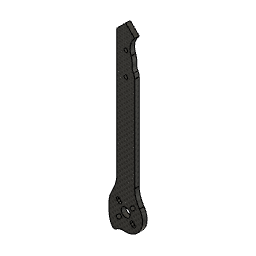
frame_arm_4mm (Autodesk Fusion 360 design; units mm, degrees)
Autodesk Fusion 360 part; units mm, degrees
sketch "Sketch3" plane through (0, 0, 0) normal (0, 0, 1) x (1, 0, 0)
  circle A0 centre (0.0083, -64.5282) radius 4.05
  circle A1 centre (0.0083, -64.5282) radius 8.75 construction
  line L0 (0.0083, -64.5282) -> (6.1955, -58.341) construction
  line L1 (0.0083, -64.5282) -> (8.7583, -64.5282) construction
  line L2 (6.4784, -60.1795) -> (8.034, -58.6238)
  arc A2 (8.034, -58.6238) -> (5.9127, -56.5025) centre (6.9733, -57.5632) ccw
  line L3 (5.9127, -56.5025) -> (4.357, -58.0581)
  arc A3 (4.357, -58.0581) -> (6.4784, -60.1795) centre (5.4177, -59.1188) ccw
  line L4 (4.357, -60.1795) -> (8.034, -56.5025) construction
  line L5 (4.357, -60.1795) -> (7.9558, -60.1795) construction
  line L6 (-4.3404, -58.0581) -> (-5.896, -56.5025)
  line L7 (-8.0173, -58.6238) -> (-6.4617, -60.1795)
  arc A4 (-6.4617, -60.1795) -> (-4.3404, -58.0581) centre (-5.401, -59.1188) ccw
  line L8 (-4.3404, -60.1795) -> (-8.0173, -56.5025) construction
  arc A5 (-5.896, -56.5025) -> (-8.0173, -58.6238) centre (-6.9567, -57.5632) ccw
  line L9 (-6.4617, -68.8769) -> (-8.0173, -70.4325)
  line L10 (-5.896, -72.5538) -> (-4.3404, -70.9982)
  arc A6 (-4.3404, -70.9982) -> (-6.4617, -68.8769) centre (-5.401, -69.9375) ccw
  line L11 (-4.3404, -68.8769) -> (-8.0173, -72.5538) construction
  arc A7 (-8.0173, -70.4325) -> (-5.896, -72.5538) centre (-6.9567, -71.4932) ccw
  line L12 (4.357, -70.9982) -> (5.9127, -72.5538)
  line L13 (8.034, -70.4325) -> (6.4784, -68.8769)
  arc A8 (6.4784, -68.8769) -> (4.357, -70.9982) centre (5.4177, -69.9375) ccw
  line L14 (4.357, -68.8769) -> (8.034, -72.5538) construction
  arc A9 (5.9127, -72.5538) -> (8.034, -70.4325) centre (6.9733, -71.4932) ccw
  circle A10 centre (0.0083, -64.5282) radius 15.1
  line L15 (-8.8515, -81.7805) -> (-9.2245, -82.0856)
  line L16 (-11.4526, -81.7512) -> (-11.2758, -81.9426)
  arc A11 (-1.4818, -79.5545) -> (-8.8515, -81.7805) centre (-2.4756, -89.5764) ccw
  line L17 (0.0083, -64.5282) -> (-15.0917, -64.5282) construction
  spline S0 degree 5 poles (-11.4526, -81.7512) (-11.5434, -81.653) (-11.7181, -81.4571) (-11.959, -81.1655) (-12.2453, -80.7768) (-12.5785, -80.2658) (-12.9207, -79.695) (-13.2839, -79.026) (-13.6569, -78.2216) (-14.017, -77.2506) (-14.3381, -76.0931) (-14.6006, -74.7468) (-14.7984, -73.2325) (-14.9351, -71.5854) (-15.0206, -69.8489) (-15.0676, -68.0675) (-15.0846, -66.6385) (-15.0904, -65.5777) (-15.0917, -64.8769) (-15.0917, -64.5282) knots 0 0 0 0 0 0 0.066667 0.133333 0.2 0.266667 0.333333 0.4 0.466667 0.533333 0.6 0.666667 0.733333 0.8 0.866667 0.933333 1 1 1 1 1 1
  arc A12 (-11.2758, -81.9426) -> (-9.2245, -82.0856) centre (-10.1742, -80.9245) ccw
  line L18 (0, 0) -> (-8.1, 0) construction
  line L19 (-8.1, 0) -> (-8.1, 74.424)
  line L20 (-8.1, 0) -> (-8.1, -40.576)
  spline S1 degree 5 poles (-15.0917, -64.5282) (-15.0917, -64.2457) (-15.0821, -63.684) (-15.0388, -62.8507) (-14.9249, -61.7598) (-14.6973, -60.4356) (-14.3963, -59.1591) (-14.0349, -57.9381) (-13.626, -56.7786) (-13.1797, -55.6822) (-12.7048, -54.6455) (-12.2091, -53.6579) (-11.7011, -52.7014) (-11.1912, -51.7478) (-10.6919, -50.7589) (-10.216, -49.6979) (-9.7711, -48.5441) (-9.3608, -47.2978) (-8.9724, -46.0117) (-8.6188, -44.7062) (-8.3284, -43.3781) (-8.1734, -42.2856) (-8.1133, -41.4415) (-8.1, -40.8665) (-8.1, -40.576) knots 0 0 0 0 0 0 0.05 0.1 0.15 0.2 0.25 0.3 0.35 0.4 0.45 0.5 0.55 0.6 0.65 0.7 0.75 0.8 0.85 0.9 0.95 1 1 1 1 1 1
  line L21 (-10.3594, -50.3117) -> (-8.6813, -45.2176)
  line L22 (-8.1, 74.424) -> (-0.039, 82.4851)
  line L23 (-8.1, 74.424) -> (3.05, 74.424) construction
  line L24 (-0.039, 82.4851) -> (8.022, 74.424)
  line L25 (-0.039, 82.4851) -> (11.1696, 82.4851) construction
  line L26 (8.022, 74.424) -> (18.0806, 64.3654) construction
  arc A13 (8.022, 74.424) -> (4.8004, 59.2677) centre (18.0806, 64.3654) ccw
  line L27 (18.0806, 64.3654) -> (8.022, 74.424) construction
  line L28 (18.0806, 64.3654) -> (4.8004, 59.2677) construction
  spline S2 degree 5 poles (4.8004, 59.2677) (4.8494, 59.1404) (4.9423, 58.8866) (5.0666, 58.5087) (5.2043, 58.0107) (5.3432, 57.4017) (5.4642, 56.809) (5.5795, 56.2321) (5.6934, 55.6644) (5.7974, 55.0914) (5.8765, 54.4957) (5.916, 53.8616) (5.9073, 53.1806) (5.8552, 52.4567) (5.782, 51.71) (5.7191, 50.9686) (5.6999, 50.2615) (5.7511, 49.6111) (5.8867, 49.0267) (6.0971, 48.4946) (6.3562, 47.9853) (6.5772, 47.5687) (6.7385, 47.238) (6.8424, 47.0077) (6.8934, 46.89) knots 0 0 0 0 0 0 0.05 0.1 0.15 0.2 0.25 0.3 0.35 0.4 0.45 0.5 0.55 0.6 0.65 0.7 0.75 0.8 0.85 0.9 0.95 1 1 1 1 1 1
  line L29 (4.1339, 60.9997) -> (5.467, 57.5357) construction
  line L30 (6.1548, 48.5926) -> (7.632, 45.1875) construction
  circle A14 centre (-0.1012, 42.8053) radius 8.1 construction
  circle A15 centre (0, 61.4851) radius 1.6
  circle A16 centre (0, 40.6251) radius 1.6
  circle A17 centre (-0.1012, 42.8053) radius 8.1
  line L31 (0, 0) -> (0, 40.6251)
  line L32 (-0.1012, 42.8053) -> (7.9988, 42.8053) construction
  line L33 (7.9988, 42.8053) -> (7.9988, -42.1947)
  arc A18 (7.9988, -42.1947) -> (12.3295, -55.799) centre (31.5321, -42.1947) ccw
  point P0 (6.1955, -58.341)
  point P1 (-6.1789, -58.341)
  point P2 (-6.1789, -58.341)
  point P3 (-6.1789, -70.7154)
  point P4 (-6.1789, -70.7154)
  point P5 (6.1955, -70.7154)
  point P6 (6.1955, -70.7154)
  point P7 (-12.7288, -80.0085)
  point P8 (-14.2896, -76.1896)
  point P9 (-13.921, -57.6445)
  point P10 (-11.7496, -52.7944)
  point P11 (-9.5204, -47.7647)
  point P12 (5.9008, 53.2841)
  point P13 (5.5742, 56.2588)
  point P14 (5.7979, 49.475)
  dimension "d1" = 8.1
  dimension "d2" = 17.5
  dimension "d3" = 45
  dimension "d4" = 5.2
  dimension "d5" = 45
  dimension "d6" = 3
  dimension "d8" = 360
  dimension "d9" = 30.2
  dimension "d10" = 1.5
  dimension "d11" = 8.1
  dimension "d12" = 115
  dimension "d13" = 45
  dimension "d14" = 11.4
  dimension "d15" = 45
  dimension "d16" = 11.4
  dimension "d17" = 14.225
  dimension "d18" = 66
  dimension "d19" = 3.2
  dimension "d20" = 21
  dimension "d21" = 3.2
  dimension "d22" = 20.86
  dimension "d23" = 16.2
  dimension "d24" = 85
  constraint concentric A0 A1
  constraint horizontal L1
  constraint coincident A0.centre A1.centre
  constraint coincident A1 P0
  constraint tangent L2 A2
  constraint tangent A2 L3
  constraint parallel L2 L3
  constraint tangent L3 A3
  constraint tangent L2 A3
  constraint midpoint A3 L4.start
  constraint midpoint A2 L4.end
  constraint coincident L0 L4.start
  constraint parallel L0 L4
  constraint midpoint L4 P0
  constraint coincident P0 L0.end
  constraint concentric A1 A10
  constraint tangent L15 A11
  constraint coincident A10 A11.start
  constraint tangent A10 A11
  constraint coincident A10 L17.end
  constraint parallel L1 L17
  constraint tangent A10 S0
  constraint tangent L15 A12
  constraint tangent L16 A12
  constraint coincident L18.start L31.start
  constraint horizontal L18
  constraint perpendicular L18 L19
  constraint perpendicular L18 L20
  constraint tangent A10 S1
  constraint midpoint P11 L21
  constraint horizontal L23
  constraint horizontal L25
  constraint perpendicular L22 L26
  constraint coincident L26.end A13.centre
  constraint coincident S2.end A14
  constraint midpoint A13.end L29
  constraint midpoint S2.end L30
  constraint coincident A16.centre L31.end
  constraint perpendicular L18 L31
  constraint coincident A14.centre A17.centre
  constraint horizontal L32
  constraint coincident A17 L32.end
  constraint coincident A14 L32.end
  constraint perpendicular L32 L33
  constraint tangent A10 A18
  constraint coincident A10 A18.end
  constraint tangent L33 A18
  measures "d1" diameter of A0
  measures "d2" diameter of A1
  measures "d3" angle of L0 L1
  measures "d4" distance of L4.start L4.end
  measures "d5" angle of L4 L5
  measures "d6" diameter of A2
  measures "d9" diameter of A10
  measures "d10" radius of A12
  measures "d11" distance of L18.start L18.end
  measures "d12" distance of L19.end L20.end
  measures "d13" angle of L22 L23
  measures "d14" distance of L19.end L22.end
  measures "d15" angle of L24 L25
  measures "d16" distance of L22.end L24.end
  measures "d17" distance of L24.end L26.end
  measures "d18" angle of L27 L28
  measures "d19" diameter of A15
  measures "d20" vertical distance of L22.end A15.centre
  measures "d21" diameter of A16
  measures "d22" distance of A15.centre A16.centre
  measures "d23" diameter of A14
  measures "d24" distance of L32.end L33.end
extrude "Extrude1" add sketch "Sketch3" along normal blind 4 contours A10 L19 L20 S1 A17 L33 A18 | A10 L15 L16 A11 S0 A12 | L19 A17 | L19 L22 L24 A13 S2 A17 picked at (-5.8704, 42.33)
equation "d2 = d1 + ( ( 2.1 * 2 ) * 1 mm ) + ( 5.2 mm )"
equation "d11 = ( 16.2 / 2 ) * 1 mm"
